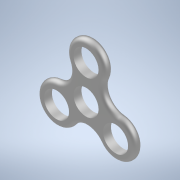
# Autodesk Inventor part: Exam 3_03-30-2022 Leo Berman
Saved by Autodesk Inventor 2022 (Build 260153000, 153)
## iProperties
Created: 2022-03-30
Part Number: Exam 3_03-30-2022 Leo Berman
Material: Aluminum 6061
Document SubType Name: Modeling
Designer: leogr
Density: 2.7 g/cm^3
Appearance: Anodized - Light Gray
Description: Al6061 Anodized Light Gray
Author: leogr
Autodesk Inventor part; units mm, degrees
ref_plane "YZ Plane" through (0, 0, 0) normal (1, 0, 0) x (0, 1, 0)
ref_plane "XZ Plane" through (0, 0, 0) normal (0, 1, 0) x (-1, 0, 0)
ref_plane "XY Plane" through (0, 0, 0) normal (0, 0, 1) x (1, 0, 0)
sketch "Sketch1" plane through (0, 0, 0) normal (0, 0, 1) x (1, 0, 0)
  circle A0 centre (0, 0) radius 11
  circle A1 centre (0, 30) radius 11
  circle A2 centre (-25.9808, -15) radius 11
  circle A3 centre (25.9808, -15) radius 11
  circle A4 centre (25.9808, -15) radius 17
  circle A5 centre (-25.9808, -15) radius 17
  circle A6 centre (0, 30) radius 17
  arc A7 (-27.6746, 1.9154) -> (-15.4961, 23.0092) centre (-29.1691, 16.8408) ccw
  arc A8 (15.4961, 23.0092) -> (27.6746, 1.9154) centre (29.1691, 16.8408) ccw
  arc A9 (12.1785, -24.9246) -> (-12.1785, -24.9246) centre (0, -33.6815) ccw
  dimension "d0" = 22
  dimension "d1" = 22
  dimension "d2" = 30
  dimension "d5" = 360
  dimension "d8" = 6
  dimension "d9" = 6
  dimension "d10" = 6
  dimension "d11" = 15
  dimension "d12" = 15
  dimension "d13" = 15
  constraints: 12 point on circle, 10 centre point, 6 tangent, 1 coincident, 1 vertical alignment, 7 other
  measures "d0" diameter of A0
  measures "d1" diameter of A1
  measures "d2" distance of A1.centre point (0, 0)
  measures "d8" radial gap between concentric circles of A3 A4
  measures "d9" radial gap between concentric circles of A2 A5
  measures "d10" radial gap between concentric circles of A1 A6
  measures "d11" radius of A7
  measures "d12" radius of A8
  measures "d13" radius of A9
extrude "Extrusion1" add sketch "Sketch1" along normal mid plane 7
full round fillet "Full Round Fillet1" first side at (17.2542, -0.5688, 3.5) centre faces at (10.4882, 43.379, 1.1667) second side at (17.2542, -0.5688, -3.5)
equation "\"d12\" = d11"
equation "\"d13\" = d11"
body "Solid1"
